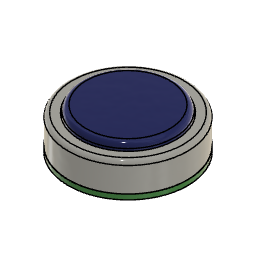
Pet_Button (Autodesk Fusion 360 design; units mm, degrees)
Autodesk Fusion 360 part; units mm, degrees
sketch "Sketch1" plane through (0, 0, 0) normal (0, 0, 1) x (1, 0, 0) in component "Button"
  circle A0 centre (0, 0) radius 14
  circle A1 centre (0, 0) radius 2.5
  arc A2 (1.5101, -15.9286) -> (-1.4866, -15.9308) centre (0.0118, -16) ccw
  arc A3 (1.5101, -15.9286) -> (-1.4866, -15.9308) centre (0, 0) ccw
  dimension "d2" = 28
  dimension "d3" = 5
  dimension "d4" = 32
  dimension "d10" = 3
  constraint coincident A0.centre A1.centre
  constraint concentric A0 A3
  constraint coincident A2.centre A3
  measures "d2" diameter of A0
  measures "d3" diameter of A1
  measures "d4" diameter of A3
  measures "d10" diameter of A2
extrude "Extrude1" add sketch "Sketch1" along normal blind 5 contours A0 | A1 makes body 1 in component "Button"
shell "Shell1" thickness 1.5 removed faces 1 at (4.6394, 2.5701, 0) on bodies 1 in component "Button"
extrude "Extrude2" add sketch "Sketch1" along normal blind 1.5 separate body contours A2 A3 makes body 2 in component "Button"
sketch "Sketch2" plane through (0, 0, 3.5) normal (0, 0, -1) x (1, 0, 0) in component "Button"
  circle A0 centre (0, 0) radius 12.5
  circle A1 centre (0, 0) radius 2.5
  dimension "d13" = 5
  constraint concentric A0 A1
  measures "d13" diameter of A1
extrude "Extrude3" add sketch "Sketch2" along normal blind 3.5 contours A1 bodies 1 in component "Button"
fillet "Fillet1" radius 1.5 1 faces at (4.6394, 2.5701, 5) on bodies 1 in component "Button"
ref_plane "WorkPlane1" through (0, 0, -5.6) normal (0, 0, 1) x (1, 0, 0) in component "Base"
sketch "Sketch1 (2)" plane through (0, 0, -5.6) normal (0, 0, 1) x (1, 0, 0) in component "Base"
  line L0 (1.5, -3) -> (-1.5, -3)
  line L1 (-3, -3) -> (-3, 3)
  line L2 (-1.5, 3) -> (1.5, 3)
  line L3 (3, 3) -> (3, -3)
  line L4 (3, -3) -> (-3, 3) construction
  line L5 (-3, -3) -> (3, 3) construction
  line L6 (-4.5, 4.5) -> (-4.5, -4.5)
  line L7 (4.5, -4.5) -> (4.5, 4.5)
  line L8 (4.5, 4.5) -> (-4.5, -4.5) construction
  line L9 (-4.5, 4.5) -> (4.5, -4.5) construction
  line L10 (-1.5, 3) -> (-1.5, 4.5)
  line L11 (0, 1.75) -> (0, 22.5)
  line L12 (1.5, 3) -> (1.5, 4.5)
  line L13 (1.75, 0) -> (22.5, 0)
  line L14 (-1.5, -3) -> (-1.5, -4.5)
  line L15 (1.5, -3) -> (1.5, -4.5)
  line L16 (-3, -3) -> (-3, -4.5)
  line L17 (-3, 3) -> (-3, 4.5)
  line L18 (3, 3) -> (3, 4.5)
  line L19 (3, -3) -> (3, -4.5)
  line L20 (-4.5, -4.5) -> (-3, -4.5)
  line L21 (-1.5, -4.5) -> (1.5, -4.5)
  line L22 (3, -4.5) -> (4.5, -4.5)
  line L23 (4.5, 4.5) -> (3, 4.5)
  line L24 (1.5, 4.5) -> (-1.5, 4.5)
  line L25 (-3, 4.5) -> (-4.5, 4.5)
  circle A0 centre (0, 0) radius 17.85
  circle A1 centre (0, 10) radius 2.1
  line L26 (-1.4252, -14.7312) -> (-1.4252, -16.2878)
  line L27 (1.4252, -14.7312) -> (1.4252, -16.2878)
  line L28 (-1.4252, 14.7312) -> (-1.4252, 16.2878)
  line L29 (1.4252, 14.7312) -> (1.4252, 16.2878)
  circle A2 centre (0, -10) radius 1.6
  circle A3 centre (-10, 0) radius 1.6
  circle A4 centre (10, 0) radius 1.6
  line L30 (-16.35, 1.4244) -> (-14.7313, 1.4244)
  line L31 (-16.35, -1.4244) -> (-14.7313, -1.4244)
  line L32 (16.35, -1.4244) -> (14.7313, -1.4244)
  line L33 (16.35, 1.4244) -> (14.7313, 1.4244)
  arc A5 (-1.4252, 14.7312) -> (-14.7313, 1.4244) centre (0, 0) ccw
  arc A6 (-14.7313, -1.4244) -> (-1.4252, -14.7312) centre (0, 0) ccw
  arc A7 (-1.4252, 16.2878) -> (-16.2878, 1.4244) centre (0, 0) ccw
  arc A8 (-16.2878, -1.4244) -> (-1.4252, -16.2878) centre (0, 0) ccw
  arc A9 (1.4252, -14.7312) -> (14.7313, -1.4244) centre (0, 0) ccw
  arc A10 (14.7313, 1.4244) -> (1.4252, 14.7312) centre (0, 0) ccw
  arc A11 (1.4252, -16.2878) -> (16.2878, -1.4244) centre (0, 0) ccw
  arc A12 (16.2878, 1.4244) -> (1.4252, 16.2878) centre (0, 0) ccw
  dimension "d21" = 32.7
  dimension "d22" = 6
  dimension "d23" = 6
  dimension "d24" = 9
  dimension "d25" = 9
  dimension "d26" = 1.5
  dimension "d37" = 29.6
  dimension "d44" = 1.5
  dimension "d45" = 4.2
  dimension "d48" = 10
  dimension "d49" = 3.2
  dimension "d50" = 10
  dimension "d51" = 3.2
  dimension "d52" = 10
  constraint coincident A0.centre A5.centre
  constraint horizontal L0
  constraint perpendicular L0 L1
  constraint parallel L0 L2
  constraint parallel L1 L3
  constraint coincident L4 A0.centre
  constraint coincident L5 A0.centre
  constraint horizontal L23
  constraint perpendicular L6 L23
  constraint parallel L20 L23
  constraint parallel L6 L7
  constraint coincident L8 A0.centre
  constraint coincident L9 A0.centre
  constraint perpendicular L2 L10
  constraint symmetric L2.start L11 L2.end
  constraint symmetric L10.end L11 L12.end
  constraint symmetric L2.start L13 L0.end
  constraint symmetric L10.end L13 L14.end
  constraint symmetric L2.end L13 L0.start
  constraint symmetric L12.end L13 L15.end
  constraint perpendicular L16 L20
  constraint coincident L17.end L23
  constraint perpendicular L17 L23
  constraint perpendicular L18 L23
  constraint coincident L19.end L20
  constraint perpendicular L19 L20
  constraint collinear L20 L21
  constraint collinear L21 L22
  constraint collinear L23 L24
  constraint collinear L24 L25
  constraint concentric A9 A11
  constraint coincident L11 A1.centre
  constraint vertical L26
  constraint symmetric L11 L26.start L27.start
  constraint symmetric L11 L26.end L27.end
  constraint symmetric L13 L26.start L28.start
  constraint symmetric L13 L26.end L28.end
  constraint symmetric L13 L27.start L29.start
  constraint symmetric L13 L27.end L29.end
  constraint concentric A7 A11
  constraint concentric A5 A9
  constraint symmetric L11 A3 A4
  constraint horizontal L30
  constraint symmetric L13 L30.start L31.start
  constraint symmetric L13 L30.end L31.end
  constraint symmetric L11 L30.start L33.start
  constraint symmetric L11 L30.end L33.end
  constraint symmetric L11 L31.start L32.start
  constraint symmetric L11 L31.end L32.end
  constraint concentric A5 A6
  constraint coincident L30 A7.end
  constraint coincident L31 A8.start
  constraint concentric A7 A8
  constraint concentric A9 A10
  constraint coincident L33 A12.start
  constraint concentric A11 A12
  constraint coincident L32 A11.end
  measures "d21" diameter of A11
  measures "d22" distance of L1.end L3.start
  measures "d23" distance of L0 L2
  measures "d24" distance of L6.end L7.start
  measures "d25" distance of L6.start L6.end
  measures "d26" distance of A0.centre L10
  measures "d37" diameter of A9
  measures "d44" distance of A0 A11
  measures "d45" diameter of A1
  measures "d48" distance of A0.centre A1.centre
  measures "d49" diameter of A2
  measures "d50" distance of A0.centre A2.centre
  measures "d51" diameter of A3
  measures "d52" distance of A0.centre A3.centre
sketch "Sketch1 (3)" plane through (0, 0, 1.5) normal (0, 0, 1) x (-1, 0, 0) in component "Cover"
  circle A0 centre (0, 0) radius 14
  arc A1 (-1.5101, 15.9286) -> (1.4866, 15.9308) centre (0, 0) ccw
  arc A2 (-1.5101, 15.9286) -> (1.4866, 15.9308) centre (-0.0118, 16) ccw
  circle A3 centre (0, 0) radius 14.3
  circle A4 centre (0, 0) radius 17.8
  arc A5 (-1.2609, 16.2512) -> (1.2372, 16.253) centre (-0.0119, 16.3) ccw
  arc A6 (-1.2609, 16.2512) -> (1.2372, 16.253) centre (0, 0) ccw
  dimension "d27" = 28.6
  dimension "d28" = 32.6
  dimension "d29" = 35.6
  dimension "d32" = 2.5
  constraint coincident A0.centre A1.centre
  constraint concentric A3 A6
  constraint concentric A4 A6
  constraint coincident A5.centre A6
  measures "d27" diameter of A3
  measures "d28" diameter of A6
  measures "d29" diameter of A4
  measures "d32" diameter of A5
extrude "Extrude1'" add sketch "Sketch1 (3)" along normal blind 1.5 separate body contours A1 A2 | A4 | A5 A6 makes body 3 in component "Cover"
extrude "Extrude2'" add sketch "Sketch1 (3)" against normal blind 7.1 contours A4 bodies 3 in component "Cover"
fillet "Fillet1'" radius 1.2 1 edges at (16.5954, 6.4368, 3) on bodies 3 in component "Cover"
combine "Combine1" operation add target body 1 tool bodies 2 in component "Button"
extrude "Extrude1''" add sketch "Sketch1 (2)" against normal blind 1.5 separate body contours L0 L14 L15 L21 | L1 L6 L16 L17 L20 L25 | L2 L10 L11 L24 | L2 L11 L12 L24 | L3 L7 L13 L18 L23 | L3 L7 L13 L19 L22 | L11 A1 | L11 A1 | L13 A4 | L13 A4 | A0 | L26 L31 A6 A8 | L27 L32 A9 A11 | L28 L30 A5 A7 | L29 L33 A10 A12 | A2 | A3 makes body 4 in component "Base"
extrude "Extrude2''" add sketch "Sketch1 (2)" along normal blind 5 contours L0 L14 L15 L21 | L1 L6 L16 L17 L20 L25 | L2 L10 L11 L24 | L2 L11 L12 L24 | L3 L7 L13 L18 L23 | L3 L7 L13 L19 L22 bodies 4 in component "Base"
extrude "Extrude3'" add sketch "Sketch1 (2)" along normal blind 4 contours L26 L31 A6 A8 | L27 L32 A9 A11 | L28 L30 A5 A7 | L29 L33 A10 A12 bodies 4 in component "Base"
extrude "Extrude4" cut sketch "Sketch1 (2)" against normal blind 5 contours L11 A1 | L11 A1 | L13 A4 | L13 A4 | A2 | A3 bodies 4 in component "Base"
sketch "Sketch1 (4)" plane through (0, 0, -5.6) normal (0, 0, 1) x (-1, 0, 0) in component "Spacer"
  circle A0 centre (-10, 0) radius 1.6
  circle A1 centre (0, 10) radius 1.6
  circle A2 centre (0, -10) radius 2.1
  circle A3 centre (10, 0) radius 1.6
  line L0 (1.4252, -16.2878) -> (1.4252, -14.7312)
  arc A4 (14.7313, 1.4244) -> (1.4252, 14.7312) centre (0, 0) ccw
  arc A5 (16.2878, 1.4244) -> (1.4252, 16.2878) centre (0, 0) ccw
  line L1 (-1.4252, 16.2878) -> (-1.4252, 14.7312)
  arc A6 (-1.4252, 14.7312) -> (-14.7313, 1.4244) centre (0, 0) ccw
  line L2 (-1.4252, -14.7312) -> (-1.4252, -16.2878)
  arc A7 (-16.2878, -1.4244) -> (-1.4252, -16.2878) centre (0, 0) ccw
  line L3 (-1.5, 3) -> (-1.5, 4.5)
  line L4 (-1.5, 4.5) -> (1.5, 4.5)
  line L5 (1.5, 4.5) -> (1.5, 3)
  line L6 (1.5, 3) -> (-1.5, 3)
  line L7 (-3, -4.5) -> (-4.5, -4.5)
  line L8 (-4.5, -4.5) -> (-4.5, 4.5)
  line L9 (-4.5, 4.5) -> (-3, 4.5)
  line L10 (-3, 4.5) -> (-3, -4.5)
  line L11 (3, 4.5) -> (4.5, 4.5)
  line L12 (4.5, 4.5) -> (4.5, -4.5)
  line L13 (4.5, -4.5) -> (3, -4.5)
  line L14 (3, -4.5) -> (3, 4.5)
  line L15 (1.5, -3) -> (1.5, -4.5)
  line L16 (1.5, -4.5) -> (-1.5, -4.5)
  line L17 (-1.5, -4.5) -> (-1.5, -3)
  line L18 (-1.5, -3) -> (1.5, -3)
  circle A8 centre (0, 0) radius 17.85
  line L19 (-2.95, -2.95) -> (2.95, -2.95)
  line L20 (2.95, -2.95) -> (2.95, 2.95)
  line L21 (2.95, 2.95) -> (-2.95, 2.95)
  line L22 (-2.95, 2.95) -> (-2.95, -2.95)
  line L23 (-2.95, -2.95) -> (2.95, 2.95) construction
  line L24 (2.95, -2.95) -> (-2.95, 2.95) construction
  line L25 (14.7313, -1.4244) -> (16.2878, -1.4244)
  arc A9 (-14.7313, -1.4244) -> (-1.4252, -14.7312) centre (0, 0) ccw
  line L26 (-16.2878, -1.4244) -> (-14.7313, -1.4244)
  line L27 (-14.7313, 1.4244) -> (-16.2878, 1.4244)
  arc A10 (-1.4252, 16.2878) -> (-16.2878, 1.4244) centre (0, 0) ccw
  line L28 (1.4252, 14.7312) -> (1.4252, 16.2878)
  line L29 (16.2878, 1.4244) -> (14.7313, 1.4244)
  arc A11 (1.4252, -14.7312) -> (14.7313, -1.4244) centre (0, 0) ccw
  arc A12 (1.4252, -16.2878) -> (16.2878, -1.4244) centre (0, 0) ccw
  dimension "d54" = 5.9
  dimension "d55" = 5.9
  constraint horizontal L19
  constraint perpendicular L19 L20
  constraint parallel L19 L21
  constraint parallel L20 L22
  constraint coincident L23 A4.centre
  constraint coincident L24 A4.centre
  constraint coincident A4.centre A5.centre
  measures "d54" distance of L20.end L21.end
  measures "d55" distance of L19.end L20.end
extrude "Extrude1'''" add sketch "Sketch1 (4)" along normal blind 0.9 separate body contours L19 L20 L21 L22 makes body 5 in component "Spacer"
sketch "Sketch1 (5)" plane through (0, 0, 1.5) normal (0, 0, 1) x (-1, 0, 0) in component "Dummy Cover"
  circle A0 centre (0, 0) radius 14
  arc A1 (-1.5101, 15.9286) -> (1.4866, 15.9308) centre (0, 0) ccw
  arc A2 (-1.5101, 15.9286) -> (1.4866, 15.9308) centre (-0.0118, 16) ccw
  circle A3 centre (0, 0) radius 14.3
  circle A4 centre (0, 0) radius 17.8
  arc A5 (-1.2609, 16.2512) -> (1.2372, 16.253) centre (-0.0119, 16.3) ccw
  arc A6 (-1.2609, 16.2512) -> (1.2372, 16.253) centre (0, 0) ccw
  dimension "d27_1" = 28.6
  dimension "d28_1" = 32.6
  dimension "d29_1" = 35.6
  dimension "d32_1" = 2.5
  constraint coincident A0.centre A1.centre
  constraint concentric A3 A6
  constraint concentric A4 A6
  constraint coincident A5.centre A6
  measures "d27_1" diameter of A3
  measures "d28_1" diameter of A6
  measures "d29_1" diameter of A4
  measures "d32_1" diameter of A5
extrude "Extrude1''''" add sketch "Sketch1 (5)" along normal blind 1.5 separate body contours A0 | A1 A2 | A3 | A4 | A5 A6 makes body 6 in component "Dummy Cover"
extrude "Extrude2'''" add sketch "Sketch1 (5)" against normal blind 6 contours A4 bodies 6 in component "Dummy Cover"
fillet "Fillet1''" radius 1.2 1 edges at (16.5954, 6.4368, 3) on bodies 6 in component "Dummy Cover"
component "Button" placed x (1, 0, 0) y (0, 1, 0) z (0, 0, 1) at (0, 0, 0)
component "Base" placed x (1, 0, 0) y (0, 1, 0) z (0, 0, 1) at (0, 0, 0)
component "Cover" placed x (1, 0, 0) y (0, 1, 0) z (0, 0, 1) at (0, 0, 0)
component "Spacer" placed x (1, 0, 0) y (0, 1, 0) z (0, 0, 1) at (0, 0, 0)
component "Dummy Cover" placed x (1, 0, 0) y (0, 1, 0) z (0, 0, 1) at (0, 0, 0)
equation "diameter = 28 mm"
equation "d2 = diameter"
equation "d4 = diameter + 2 * lip"
equation "d5 = button_height"
equation "d7 = button_wall"
equation "button_height = 5 mm"
equation "button_wall = 1.5 mm"
equation "d10 = lip * 2 - 1 mm"
equation "d11 = button_wall"
equation "d14 = button_height - button_wall"
equation "d18 = -( stop_height + 1.6 mm )"
equation "lip = 2 mm"
equation "clearance = 0.3 mm"
equation "d21 = diameter + 2 * ( lip + clearance ) + 0.1 mm"
equation "d24 = 6 mm + 3 mm"
equation "d25 = 6 mm + 3 mm"
equation "d27 = diameter + 2 * clearance"
equation "d28 = diameter + 2 * ( lip + clearance )"
equation "d29 = diameter + 2 * ( lip + clearance + button_wall )"
equation "d30 = button_wall"
equation "d33 = -( stop_height + 3.1 mm )"
equation "d37 = diameter + 2 * ( lip + clearance - button_wall )"
equation "d38 = -button_wall"
equation "d40 = button_height"
equation "d42 = stop_height"
equation "d44 = button_wall"
equation "stop_height = 4 mm"
equation "d27_1 = diameter + 2 * clearance"
equation "d28_1 = diameter + 2 * ( lip + clearance )"
equation "d29_1 = diameter + 2 * ( lip + clearance + button_wall )"
equation "d30_1 = button_wall"
equation "d33_1 = -( stop_height + 2 mm )"
